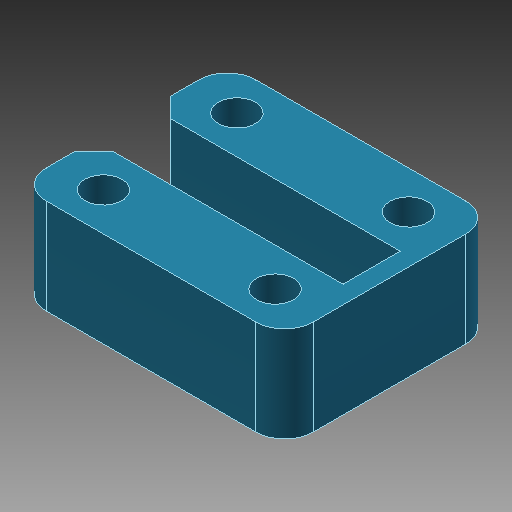
# Autodesk Inventor part: Фиксатор_сервопривода
Saved by Autodesk Inventor 2021.3 (Build 253353000, 353)
## iProperties
RuleStatus: InUse
Part Number: Фиксатор_сервопривода
Checked By: Якушев
Engr Approved By: Малов
Material: По умолчанию1
Document SubType Name: Modeling
Mfg Approved By: Судаков
Designer: Смирнов
Density: 1 g/cm^3
Appearance: Бирюзовый
AfterMaterialChange0: Материал
BeforeDocSave0: Материал
AfterAnyiPropertyChange0: Материал
Материал: По умолчанию1
Author: Смирнов
Autodesk Inventor part; units mm, degrees
ref_plane "YZ Plane" through (0, 0, 0) normal (1, 0, 0) x (0, 1, 0)
ref_plane "XZ Plane" through (0, 0, 0) normal (0, 1, 0) x (-1, 0, 0)
ref_plane "РабПлоскость1" through (-243.8305, -139, 0) normal (0, 1, 0) x (-1, 0, 0)
sketch "Эскиз1" plane through (-243.8305, -139, 0) normal (0, 1, 0) x (-1, 0, 0)
  line L0 (-217.7305, 128) -> (-241.9805, 128) projected
  line L1 (-241.9805, 128) -> (-241.9805, 134) projected
  line L2 (-217.7305, 134) -> (-241.9805, 134) projected
  line L3 (-217.7305, 128) -> (-217.7305, 134) construction
  line L4 (-218.8555, 120) -> (-240.8555, 120)
  line L5 (-243.8555, 123) -> (-243.8555, 139)
  line L6 (-240.8555, 142) -> (-218.8555, 142)
  line L7 (-215.8555, 139) -> (-215.8555, 123)
  line L8 (-229.8555, 128) -> (-229.8555, 134) construction
  line L9 (-217.7305, 131) -> (-241.9805, 131) construction
  line L10 (-238.8555, 138) -> (-220.8555, 138) construction
  line L11 (-220.8555, 138) -> (-220.8555, 124) construction
  line L12 (-220.8555, 124) -> (-238.8555, 124) construction
  line L13 (-238.8555, 124) -> (-238.8555, 138) construction
  line L14 (-238.8555, 138) -> (-220.8555, 124) construction
  line L15 (-220.8555, 138) -> (-238.8555, 124) construction
  circle A0 centre (-220.8555, 124) radius 1.95
  circle A1 centre (-238.8555, 124) radius 1.95
  circle A2 centre (-238.8555, 138) radius 1.95
  circle A3 centre (-220.8555, 138) radius 1.95
  arc A4 (-218.8555, 120) -> (-215.8555, 123) centre (-218.8555, 123) ccw
  arc A5 (-215.8555, 139) -> (-218.8555, 142) centre (-218.8555, 139) ccw
  arc A6 (-240.8555, 142) -> (-243.8555, 139) centre (-240.8555, 139) ccw
  arc A7 (-243.8555, 123) -> (-240.8555, 120) centre (-240.8555, 123) ccw
  line L16 (-217.7305, 128) -> (-215.8555, 128)
  line L17 (-215.8555, 128) -> (-215.8555, 134)
  line L18 (-215.8555, 134) -> (-217.7305, 134)
  line L19 (-217.7305, 134) -> (-217.7305, 128) construction
  point P0 (-243.8305, 0)
  point P1 (-243.8555, 142)
  point P2 (-243.8555, 120)
  point P3 (-215.8555, 142)
  point P4 (-229.8555, 131)
  dimension "d0" = 28
  dimension "d1" = 22
  dimension "d2" = 3.9
  dimension "d3" = 18
  dimension "d4" = 14
  dimension "d5" = 3
  constraints: 32 end point, 8 centre point, 8 point on circle, 8 tangent, 7 midpoint, 7 point on line, 6 equal radius, 6 parallel, 4 coincident, 3 horizontal, 3 perpendicular, 1 collinear, 2 other
  measures "d0" distance of point (-243.855, 142) point (-215.855, 142)
  measures "d1" distance of point (-243.855, 120) point (-243.855, 142)
  measures "d2" diameter of A0
  measures "d3" distance of L11.end L12.end
  measures "d4" distance of L12.end L10.start
  measures "d5" radius of A4
extrude "Выдавливание1" add sketch "Эскиз1" along normal blind 10 contours L16 L7 A4 L4 A7 L5 A6 L6 A5 L18 L2 L1 L0
chamfer "Фаска1" distance 2 angle 45 2 edges at (-27.975, -134, 134) (-27.975, -134, 128)
